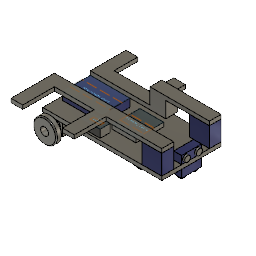
Party Crasher v9 (Autodesk Fusion 360 design; units mm, degrees)
Autodesk Fusion 360 part; units mm, degrees
sketch "Sketch1" plane through (0, 0, 0) normal (0, 0, 1) x (1, 0, 0)
  line L0 (0, 0) -> (300, 0)
  line L1 (300, 0) -> (300, 150)
  line L2 (300, 150) -> (0, 150)
  line L3 (0, 150) -> (0, 0)
  constraint horizontal L0
  constraint vertical L1
  constraint horizontal L2
  constraint vertical L3
  constraint coincident L0.start L3.end
extrude "Extrude1" add sketch "Sketch1" along normal blind 10 makes body 1
move_body "Move1" bodies 1 to x (1, 0, 0) y (0, 1, 0) z (0, 0, 1) at (0, 0, 50)
copy_body "Body->Comp1" bodies 1 removing the originals makes body 2 in component "Base"
sketch "Sketch1 (2)" plane through (0, 0, 60) normal (0, 0, 1) x (-1, 0, 0) in component "Arms"
  line L0 (0, -150) -> (0, 0)
  line L1 (0, 0) -> (-300, 0)
  line L2 (-300, 0) -> (-300, -150)
  line L3 (-300, -150) -> (0, -150)
  line L4 (-300, 0) -> (-250, 0)
  line L5 (-250, 0) -> (-250, -30)
  line L6 (-250, -30) -> (-300, -30)
  line L7 (-300, -30) -> (-300, 0)
  line L8 (-300, -150) -> (-250, -150)
  line L9 (-250, -150) -> (-250, -120)
  line L10 (-250, -120) -> (-300, -120)
  line L11 (-300, -120) -> (-300, -150)
  constraint horizontal L4
  constraint vertical L5
  constraint horizontal L6
  constraint vertical L7
  constraint coincident L1.end L2.start
  constraint horizontal L8
  constraint vertical L9
  constraint horizontal L10
  constraint vertical L11
  constraint coincident L2.end L3.start
extrude "Extrude1'" add sketch "Sketch1 (2)" along normal blind 50 separate body contours L2 L3 L8 L9 L10 L11 | L1 L2 L4 L5 L6 L7 makes body 3 at (283.3333, 150, 76.6667) makes body 4 at (266.6667, 30, 76.6667) in component "Arms"
sketch "Sketch2" plane through (0, 0, 110) normal (0, 0, 1) x (-1, 0, 0) in component "Arms"
  line L0 (-300, -30) -> (-250, -30)
  line L1 (-250, -30) -> (-250, 0)
  line L2 (-250, 0) -> (-300, 0)
  line L3 (-300, 0) -> (-300, -30)
  line L4 (-300, 0) -> (0, 0)
  line L5 (0, 0) -> (0, -30)
  line L6 (0, -30) -> (-300, -30)
  line L7 (-300, -30) -> (-300, 0)
  constraint horizontal L4
  constraint vertical L5
  constraint horizontal L6
  constraint vertical L7
  constraint coincident L2.end L3.start
sketch "Sketch10" plane through (0, 0, 110) normal (0, 0, 1) x (-1, 0, 0) in component "Arms"
  line L0 (-300, -30) -> (-250, -30)
  line L1 (-250, -30) -> (-250, 0)
  line L2 (-250, 0) -> (-300, 0)
  line L3 (-300, 0) -> (-300, -30)
  line L4 (-300, 0) -> (0, 0)
  line L5 (0, 0) -> (0, -30)
  line L6 (0, -30) -> (-300, -30)
  line L7 (-300, -30) -> (-300, 0)
  constraint horizontal L4
  constraint vertical L5
  constraint horizontal L6
  constraint vertical L7
  constraint coincident L2.end L3.start
extrude "Extrude1''" add sketch "Sketch10" along normal blind 10 separate body makes body 5 in component "Right Arm"
move_body "Move1'" bodies 5 to x (1, 0, 0) y (0, 1, 0) z (0, 0, 1) at (0, 0, 10) in component "Right Arm"
sketch "Sketch15" plane through (0, 0, 0) normal (0, -1, 0) x (1, 0, 0) in component "Arms"
  line L0 (0, 120) -> (300, 120)
  line L1 (300, 120) -> (300, 130)
  line L2 (300, 130) -> (0, 130)
  line L3 (0, 130) -> (0, 120)
  line L4 (0, 120) -> (30, 120)
  line L5 (30, 120) -> (30, 130)
  line L6 (30, 130) -> (0, 130)
  line L7 (0, 130) -> (0, 120)
  line L8 (160, 120) -> (130, 120)
  line L9 (130, 120) -> (130, 130)
  line L10 (130, 130) -> (160, 130)
  line L11 (160, 130) -> (160, 120)
  constraint horizontal L4
  constraint vertical L5
  constraint horizontal L6
  constraint vertical L7
  constraint coincident L2 L5.end
  constraint coincident L0.start L3.end
  constraint horizontal L8
  constraint vertical L9
  constraint horizontal L10
  constraint vertical L11
  constraint coincident L2 L9.end
  constraint coincident L0 L8.start
sketch "Sketch1 (3)" plane through (0, 0, 0) normal (0, -1, 0) x (1, 0, 0) in component "Right Arm"
  line L0 (0, 120) -> (300, 120)
  line L1 (300, 120) -> (300, 130)
  line L2 (300, 130) -> (0, 130)
  line L3 (0, 130) -> (0, 120)
  line L4 (0, 120) -> (30, 120)
  line L5 (30, 120) -> (30, 130)
  line L6 (30, 130) -> (0, 130)
  line L7 (0, 130) -> (0, 120)
  line L8 (160, 120) -> (130, 120)
  line L9 (130, 120) -> (130, 130)
  line L10 (130, 130) -> (160, 130)
  line L11 (160, 130) -> (160, 120)
  constraint horizontal L4
  constraint vertical L5
  constraint horizontal L6
  constraint vertical L7
  constraint coincident L2 L5.end
  constraint coincident L0.start L3.end
  constraint horizontal L8
  constraint vertical L9
  constraint horizontal L10
  constraint vertical L11
  constraint coincident L2 L9.end
  constraint coincident L0 L8.start
extrude "Extrude2" add sketch "Sketch1 (3)" along normal blind 80 contours L0 L2 L3 L4 L5 L6 L7 | L0 L2 L8 L9 L10 L11 bodies 5 in component "Right Arm"
move_body "Move3" bodies 5 to x (1, 0, 0) y (0, 1, 0) z (0, 0, 1) at (0, 0, -10) in component "Right Arm"
sketch "Sketch16" plane through (0, 0, 110) normal (0, 0, 1) x (-1, 0, 0) in component "Arms"
  line L0 (-300, -120) -> (-300, -150)
  line L1 (-300, -150) -> (-250, -150)
  line L2 (-250, -150) -> (-250, -120)
  line L3 (-250, -120) -> (-300, -120)
  line L4 (-300, -120) -> (-150, -120)
  line L5 (-150, -120) -> (-150, -150)
  line L6 (-150, -150) -> (-300, -150)
  line L7 (-300, -150) -> (-300, -120)
  constraint horizontal L4
  constraint vertical L5
  constraint horizontal L6
  constraint vertical L7
  constraint coincident L0.start L3.end
extrude "Extrude1'''" add sketch "Sketch16" along normal blind 10 separate body makes body 6 in component "Right Arm (1)"
sketch "Sketch17" plane through (0, 0, 110) normal (0, 0, -1) x (1, 0, 0) in component "Arms"
  line L0 (150, -150) -> (300, -150)
  line L1 (300, -150) -> (300, -120)
  line L2 (300, -120) -> (150, -120)
  line L3 (150, -120) -> (150, -150)
  line L4 (200, -150) -> (150, -150)
  line L5 (150, -150) -> (150, -120)
  line L6 (150, -120) -> (200, -120)
  line L7 (200, -120) -> (200, -150)
  constraint horizontal L4
  constraint vertical L5
  constraint horizontal L6
  constraint vertical L7
  constraint coincident L2.end L3.start
  constraint coincident L0 L4.start
sketch "Sketch18" plane through (0, 0, 100) normal (0, 0, -1) x (1, 0, 0) in component "Arms"
  line L0 (200, -120) -> (150, -120)
  line L1 (150, -120) -> (150, -150)
  line L2 (150, -150) -> (200, -150)
  line L3 (200, -150) -> (200, -120)
  line L4 (200, -150) -> (0, -150)
  line L5 (0, -150) -> (0, -120)
  line L6 (0, -120) -> (200, -120)
  line L7 (200, -120) -> (200, -150)
  constraint horizontal L4
  constraint vertical L5
  constraint horizontal L6
  constraint vertical L7
  constraint coincident L2.end L3.start
sketch "Sketch1 (4)" plane through (0, 0, 110) normal (0, 0, -1) x (1, 0, 0) in component "Right Arm (1)"
  line L0 (150, -150) -> (300, -150)
  line L1 (300, -150) -> (300, -120)
  line L2 (300, -120) -> (150, -120)
  line L3 (150, -120) -> (150, -150)
  line L4 (190, -150) -> (150, -150)
  line L5 (150, -150) -> (150, -120)
  line L6 (150, -120) -> (190, -120)
  line L7 (190, -120) -> (190, -150)
  constraint horizontal L4
  constraint vertical L5
  constraint horizontal L6
  constraint vertical L7
  constraint coincident L2.end L3.start
  constraint coincident L0 L4.start
extrude "Extrude2'" add sketch "Sketch1 (4)" along normal blind 30 contours L0 L2 L3 L4 L5 L6 L7 bodies 6 in component "Right Arm (1)"
sketch "Sketch2 (2)" plane through (0, 0, 80) normal (0, 0, -1) x (1, 0, 0) in component "Right Arm (1)"
  line L0 (190, -120) -> (150, -120)
  line L1 (150, -120) -> (150, -150)
  line L2 (150, -150) -> (190, -150)
  line L3 (190, -150) -> (190, -120)
  line L4 (190, -120) -> (0, -120)
  line L5 (0, -120) -> (0, -150)
  line L6 (0, -150) -> (190, -150)
  line L7 (190, -150) -> (190, -120)
  constraint horizontal L4
  constraint vertical L5
  constraint horizontal L6
  constraint vertical L7
  constraint coincident L0.start L3.end
extrude "Extrude3" add sketch "Sketch2 (2)" along normal blind 10 bodies 6 in component "Right Arm (1)"
move_body "Move1''" bodies 6 to x (1, 0, 0) y (0, 1, 0) z (0, 0, 1) at (0, 0, 20) in component "Right Arm (1)"
move_body "Move2" bodies 6 to x (1, 0, 0) y (0, 1, 0) z (0, 0, 1) at (0, 0, -20) in component "Right Arm (1)"
sketch "Sketch4" plane through (0, 150, 0) normal (0, 1, 0) x (-1, 0, 0) in component "Right Arm (1)"
  line L0 (-150, 80) -> (-150, 120)
  line L1 (-150, 120) -> (-300, 120)
  line L2 (-300, 120) -> (-300, 110)
  line L3 (-300, 110) -> (-190, 110)
  line L4 (-190, 110) -> (-190, 70)
  line L5 (-190, 70) -> (0, 70)
  line L6 (0, 70) -> (0, 80)
  line L7 (0, 80) -> (-150, 80)
  line L8 (0, 70) -> (-30, 70)
  line L9 (-30, 70) -> (-30, 80)
  line L10 (-30, 80) -> (0, 80)
  line L11 (0, 80) -> (0, 70)
  line L12 (-150, 70) -> (-120, 70)
  line L13 (-120, 70) -> (-120, 80)
  line L14 (-120, 80) -> (-150, 80)
  line L15 (-150, 80) -> (-150, 70)
  constraint horizontal L8
  constraint vertical L9
  constraint horizontal L10
  constraint vertical L11
  constraint coincident L7 L9.end
  constraint coincident L5.end L6.start
  constraint horizontal L12
  constraint vertical L13
  constraint horizontal L14
  constraint vertical L15
  constraint coincident L7 L13.end
  constraint coincident L5 L12.start
extrude "Extrude4" add sketch "Sketch4" along normal blind 60 contours L5 L7 L12 L13 L14 L15 | L5 L6 L7 L8 L9 L10 L11 bodies 6 in component "Right Arm (1)"
sketch "Sketch4 (2)" plane through (0, 0, 50) normal (0, 0, -1) x (1, 0, 0)
  line L0 (0, 0) -> (0, -150)
  line L1 (0, -150) -> (300, -150)
  line L2 (300, -150) -> (300, 0)
  line L3 (300, 0) -> (0, 0)
  line L4 (300, -75) -> (150, -75) construction
  line L5 (300, -75) -> (280, -75)
  line L6 (280, -75) -> (280, -100)
  line L7 (280, -100) -> (300, -100)
  line L8 (300, -100) -> (300, -75)
  line L9 (280, -75) -> (300, -75)
  line L10 (300, -75) -> (300, -50)
  line L11 (300, -50) -> (280, -50)
  line L12 (280, -50) -> (280, -75)
  constraint midpoint L2 L4.start
  constraint perpendicular L2 L4
  constraint horizontal L5
  constraint vertical L6
  constraint horizontal L7
  constraint vertical L8
  constraint horizontal L9
  constraint vertical L10
  constraint horizontal L11
  constraint vertical L12
  constraint coincident L2 L10.end
extrude "Extrude1''''" add sketch "Sketch4 (2)" along normal blind 20 separate body contours L2 L5 L9 L10 L11 L12 | L2 L5 L6 L7 L8 L9 makes body 7 in component "Ultrasonic Sensor"
sketch "Sketch5" plane through (300, 0, 0) normal (1, 0, 0) x (0, 1, 0)
  line L0 (100, 50) -> (50, 50)
  line L1 (50, 50) -> (50, 30)
  line L2 (50, 30) -> (100, 30)
  line L3 (100, 30) -> (100, 50)
  circle A0 centre (60, 40) radius 7.2433
  circle A1 centre (90, 40) radius 7.4829
extrude "Extrude2''" add sketch "Sketch5" along normal blind 5 contours A0 | A1 bodies 7 in component "Ultrasonic Sensor"
move_body "Move1'''" bodies 7 to x (1, 0, 0) y (0, 1, 0) z (0, 0, 1) at (0, 0, 30) in component "Ultrasonic Sensor"
copy_body "CopyPasteBodies1" bodies 7 makes body 8
move_body "Move2'" bodies 8 to x (0, 0, -1) y (0, 1, 0) z (1, 0, 0) at (220, 0, 330)
sketch "Sketch6" plane through (0, 0, 60) normal (0, 0, 1) x (-1, 0, 0)
  line L0 (0, -150) -> (0, 0)
  line L1 (0, 0) -> (-300, 0)
  line L2 (-300, 0) -> (-300, -150)
  line L3 (-300, -150) -> (0, -150)
  line L4 (-10, -110) -> (-110, -110)
  line L5 (-110, -110) -> (-110, -40)
  line L6 (-110, -40) -> (-10, -40)
  line L7 (-10, -40) -> (-10, -110)
  constraint horizontal L4
  constraint vertical L5
  constraint horizontal L6
  constraint vertical L7
extrude "Extrude1'''''" add sketch "Sketch6" along normal blind 20 contours L4 L5 L6 L7 bodies 2 in component "Base"
sketch "Sketch7" plane through (0, 0, 60) normal (0, 0, 1) x (-1, 0, 0)
  line L0 (-10, -40) -> (-10, -110)
  line L1 (-10, -110) -> (-110, -110)
  line L2 (-110, -110) -> (-110, -40)
  line L3 (-110, -40) -> (-10, -40)
  line L4 (0, -150) -> (0, 0)
  line L5 (0, 0) -> (-300, 0)
  line L6 (-300, 0) -> (-300, -150)
  line L7 (-300, -150) -> (0, -150)
  line L8 (-135, -110) -> (-195, -110)
  line L9 (-195, -110) -> (-195, -40)
  line L10 (-195, -40) -> (-135, -40)
  line L11 (-135, -40) -> (-135, -110)
  constraint horizontal L8
  constraint vertical L9
  constraint horizontal L10
  constraint vertical L11
extrude "Extrude2'''" add sketch "Sketch7" along normal blind 10 contours L8 L9 L10 L11 bodies 2 in component "Base"
sketch "Sketch8" plane through (0, 0, 80) normal (0, 0, 1) x (-1, 0, 0)
  line L0 (-10, -40) -> (-110, -40)
  line L1 (-110, -40) -> (-110, -110)
  line L2 (-110, -110) -> (-10, -110)
  line L3 (-10, -110) -> (-10, -40)
  line L4 (-10, -59.9864) -> (-110, -59.9864) construction
  line L5 (-110, -59.9864) -> (-110, -90.0136) construction
  line L6 (-110, -90.0136) -> (-10, -90.0136) construction
  line L7 (-10, -90.0136) -> (-10, -59.9864) construction
  dimension "d72" = 5
  constraint midpoint L1
  constraint midpoint L3
sketch "Sketch9" plane through (0, 0, 70) normal (0, 0, 1) x (-1, 0, 0)
  line L0 (-135, -40) -> (-195, -40)
  line L1 (-195, -40) -> (-195, -110)
  line L2 (-195, -110) -> (-135, -110)
  line L3 (-135, -110) -> (-135, -40)
  line L4 (-135, -60) -> (-195, -60) construction
  line L5 (-195, -60) -> (-195, -85) construction
  line L6 (-195, -85) -> (-135, -85) construction
  line L7 (-135, -85) -> (-135, -60) construction
  dimension "d73" = 5
  constraint coincident L1
sketch "Sketch10 (2)" plane through (0, 0, 60) normal (0, 0, 1) x (-1, 0, 0)
  line L0 (-135, -40) -> (-135, -110)
  line L1 (-135, -110) -> (-195, -110)
  line L2 (-195, -110) -> (-195, -40)
  line L3 (-195, -40) -> (-135, -40)
  line L4 (-10, -40) -> (-10, -110)
  line L5 (-10, -110) -> (-110, -110)
  line L6 (-110, -110) -> (-110, -40)
  line L7 (-110, -40) -> (-10, -40)
  line L8 (0, -150) -> (0, 0)
  line L9 (0, 0) -> (-300, 0)
  line L10 (-300, 0) -> (-300, -150)
  line L11 (-300, -150) -> (0, -150)
  line L12 (-95, -30) -> (-140, -30)
  line L13 (-140, -30) -> (-140, -5)
  line L14 (-140, -5) -> (-95, -5)
  line L15 (-95, -5) -> (-95, -30)
  constraint horizontal L12
  constraint vertical L13
  constraint horizontal L14
  constraint vertical L15
extrude "Extrude3'" add sketch "Sketch10 (2)" along normal blind 20 contours L12 L13 L14 L15 bodies 2 in component "Base"
sketch "Sketch11" plane through (0, 0, 80) normal (0, 0, 1) x (-1, 0, 0)
  line L0 (-95, -5) -> (-140, -5)
  line L1 (-140, -5) -> (-140, -30)
  line L2 (-140, -30) -> (-95, -30)
  line L3 (-95, -30) -> (-95, -5)
  line L4 (-106, -14) -> (-131, -14) construction
  line L5 (-131, -14) -> (-131, -23) construction
  line L6 (-131, -23) -> (-106, -23) construction
  line L7 (-106, -23) -> (-106, -14) construction
  dimension "d76" = 4
sketch "Sketch14" plane through (0, 0, 50) normal (0, 0, -1) x (1, 0, 0)
  line L0 (0, 0) -> (0, -150)
  line L1 (0, -150) -> (300, -150)
  line L2 (300, -150) -> (300, 0)
  line L3 (300, 0) -> (0, 0)
  line L4 (10, -10) -> (40, -10)
  line L5 (40, -10) -> (40, -20)
  line L6 (40, -20) -> (10, -20)
  line L7 (10, -20) -> (10, -10)
  line L8 (10, -140) -> (40, -140)
  line L9 (40, -140) -> (40, -130)
  line L10 (40, -130) -> (10, -130)
  line L11 (10, -130) -> (10, -140)
  constraint horizontal L4
  constraint vertical L5
  constraint horizontal L6
  constraint vertical L7
  constraint horizontal L8
  constraint vertical L9
  constraint horizontal L10
  constraint vertical L11
extrude "Extrude5" add sketch "Sketch14" along normal blind 40 contours L4 L5 L6 L7 | L8 L9 L10 L11 bodies 2 in component "Base"
sketch "Sketch1 (5)" plane through (0, 10, 0) normal (0, -1, 0) x (1, 0, 0) in component "Base"
  line L0 (40, 50) -> (10, 50)
  line L1 (10, 50) -> (10, 10)
  line L2 (10, 10) -> (40, 10)
  line L3 (40, 10) -> (40, 50)
  circle A0 centre (25, 30) radius 10
extrude "Extrude6" add sketch "Sketch1 (5)" along normal blind 15 contours A0 bodies 2 in component "Base"
sketch "Sketch2 (3)" plane through (0, -5, 0) normal (0, -1, 0) x (1, 0, 0) in component "Base"
  circle A0 centre (25, 30) radius 10
  circle A1 centre (25, 30) radius 30
  constraint concentric A0 A1
extrude "Extrude1''''''" add sketch "Sketch2 (3)" along normal blind 15 separate body makes body 9 in component "Component"
fillet "Fillet1" radius 2.5 2 edges at (-2.9698, -20, 19.1515) (-2.9698, -5, 19.1515) on bodies 9 in component "Component"
sketch "Sketch3" plane through (0, 140, 0) normal (0, 1, 0) x (-1, 0, 0) in component "Base"
  line L0 (-10, 50) -> (-40, 50)
  line L1 (-40, 50) -> (-40, 10)
  line L2 (-40, 10) -> (-10, 10)
  line L3 (-10, 10) -> (-10, 50)
  circle A0 centre (-25, 25) radius 10
extrude "Extrude7" add sketch "Sketch3" along normal blind 15 contours A0 bodies 2 in component "Base"
sketch "Sketch4 (3)" plane through (0, 155, 0) normal (0, 1, 0) x (-1, 0, 0) in component "Base"
  circle A0 centre (-25, 25) radius 10
  circle A1 centre (-25, 25) radius 30
  constraint concentric A0 A1
extrude "Extrude1'''''''" add sketch "Sketch4 (3)" along normal blind 15 separate body makes body 10 in component "Component'"
fillet "Fillet1'" radius 2.5 2 edges at (52.9698, 170, 14.1515) (52.9698, 155, 14.1515) on bodies 10 in component "Component'"
sketch "Sketch5 (2)" plane through (0, 0, 50) normal (0, 0, -1) x (1, 0, 0) in component "Base"
  line L0 (10, -130) -> (40, -130)
  line L1 (40, -130) -> (40, -140)
  line L2 (40, -140) -> (10, -140)
  line L3 (10, -140) -> (10, -130)
  line L4 (10, -20) -> (10, -10)
  line L5 (10, -10) -> (40, -10)
  line L6 (40, -10) -> (40, -20)
  line L7 (40, -20) -> (10, -20)
  line L8 (0, 0) -> (0, -150)
  line L9 (0, -150) -> (300, -150)
  line L10 (300, -150) -> (300, 0)
  line L11 (300, 0) -> (0, 0)
  line L12 (0, -75) -> (300, -75) construction
  line L13 (180, -70) -> (210, -70)
  line L14 (210, -70) -> (210, -60)
  line L15 (210, -60) -> (180, -60)
  line L16 (180, -60) -> (180, -70)
  line L17 (180, -80) -> (210, -80)
  line L18 (210, -80) -> (210, -90)
  line L19 (210, -90) -> (180, -90)
  line L20 (180, -90) -> (180, -80)
  constraint midpoint L8 L12.start
  constraint midpoint L10 L12.end
  constraint horizontal L13
  constraint vertical L14
  constraint horizontal L15
  constraint vertical L16
  constraint horizontal L17
  constraint vertical L18
  constraint horizontal L19
  constraint vertical L20
extrude "Extrude8" add sketch "Sketch5 (2)" along normal blind 40 contours L13 L14 L15 L16 | L17 L18 L19 L20 bodies 2 in component "Base"
sketch "Sketch6 (2)" plane through (0, 60, 0) normal (0, -1, 0) x (1, 0, 0) in component "Base"
  line L0 (210, 50) -> (180, 50)
  line L1 (180, 50) -> (180, 10)
  line L2 (180, 10) -> (210, 10)
  line L3 (210, 10) -> (210, 50)
  circle A0 centre (195, 25) radius 10
extrude "Extrude9" add sketch "Sketch6 (2)" along normal blind 5 contours A0 bodies 2 in component "Base"
sketch "Sketch7 (2)" plane through (0, 55, 0) normal (0, -1, 0) x (1, 0, 0) in component "Base"
  circle A0 centre (195, 25) radius 10
  circle A1 centre (195, 25) radius 25
  constraint concentric A0 A1
extrude "Extrude1''''''''" add sketch "Sketch7 (2)" along normal blind 10 separate body makes body 11 in component "Component''"
fillet "Fillet1''" radius 2.5 2 edges at (171.6918, 45, 15.9596) (171.6918, 55, 15.9596) on bodies 11 in component "Component''"
sketch "Sketch8 (2)" plane through (0, 90, 0) normal (0, 1, 0) x (-1, 0, 0) in component "Base"
  line L0 (-180, 50) -> (-210, 50)
  line L1 (-210, 50) -> (-210, 10)
  line L2 (-210, 10) -> (-180, 10)
  line L3 (-180, 10) -> (-180, 50)
  circle A0 centre (-195, 25) radius 9.8182
extrude "Extrude10" add sketch "Sketch8 (2)" along normal blind 5 contours A0 bodies 2 in component "Base"
sketch "Sketch9 (2)" plane through (0, 95, 0) normal (0, 1, 0) x (-1, 0, 0) in component "Base"
  circle A0 centre (-195, 25) radius 9.8182
  circle A1 centre (-195, 25) radius 25
  constraint concentric A0 A1
extrude "Extrude1'''''''''" add sketch "Sketch9 (2)" along normal blind 10 separate body makes body 12 in component "Component'''"
fillet "Fillet1'''" radius 2.5 2 edges at (218.3082, 105, 15.9596) (218.3082, 95, 15.9596) on bodies 12 in component "Component'''"
sketch "Sketch10 (3)" plane through (0, 0, 50) normal (0, 0, -1) x (1, 0, 0) in component "Base"
  line L0 (180, -90) -> (180, -80)
  line L1 (180, -80) -> (210, -80)
  line L2 (210, -80) -> (210, -90)
  line L3 (210, -90) -> (180, -90)
  line L4 (180, -60) -> (210, -60)
  line L5 (210, -60) -> (210, -70)
  line L6 (210, -70) -> (180, -70)
  line L7 (180, -70) -> (180, -60)
  line L8 (10, -130) -> (40, -130)
  line L9 (40, -130) -> (40, -140)
  line L10 (40, -140) -> (10, -140)
  line L11 (10, -140) -> (10, -130)
  line L12 (10, -20) -> (10, -10)
  line L13 (10, -10) -> (40, -10)
  line L14 (40, -10) -> (40, -20)
  line L15 (40, -20) -> (10, -20)
  line L16 (0, 0) -> (0, -150)
  line L17 (0, -150) -> (300, -150)
  line L18 (300, -150) -> (300, 0)
  line L19 (300, 0) -> (0, 0)
  line L20 (140, -40) -> (40, -40)
  line L21 (40, -40) -> (40, -110)
  line L22 (40, -110) -> (140, -110)
  line L23 (140, -110) -> (140, -40)
  constraint horizontal L20
  constraint vertical L21
  constraint horizontal L22
  constraint vertical L23
extrude "Extrude11" add sketch "Sketch10 (3)" along normal blind 20 contours L20 L21 L22 L23 bodies 2 in component "Base"
component "Base" placed x (1, 0, 0) y (0, 1, 0) z (0, 0, 1) at (0, 0, 0)
component "Arms" placed x (1, 0, 0) y (0, 1, 0) z (0, 0, 1) at (0, 0, 0)
component "Ultrasonic Sensor" placed x (1, 0, 0) y (0, 1, 0) z (0, 0, 1) at (0, 0, 0)
component "Component" placed x (1, 0, 0) y (0, 1, 0) z (0, 0, 1) at (0, 0, 0) in component "Base"
component "Component'" placed x (1, 0, 0) y (0, 1, 0) z (0, 0, 1) at (0, 0, 0) in component "Base"
component "Component''" placed x (1, 0, 0) y (0, 1, 0) z (0, 0, 1) at (0, 0, 0) in component "Base"
component "Component'''" placed x (1, 0, 0) y (0, 1, 0) z (0, 0, 1) at (0, 0, 0) in component "Base"
component "Right Arm" placed x (1, 0, 0) y (0, 1, 0) z (0, 0, 1) at (0, 0, 0) in component "Arms"
component "Right Arm (1)" placed x (1, 0, 0) y (0, 1, 0) z (0, 0, 1) at (0, 0, 0) in component "Arms"
